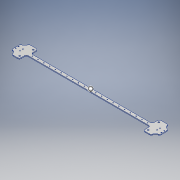
# Autodesk Inventor part: XY_Plate
Saved by Autodesk Inventor 2019 (Build 230136000, 136)
## iProperties
Created: 2018-10-13
Part Number: XY_Plate
Material: Aluminum 6061
Document SubType Name: Sheet Metal
Designer: Ax
Density: 2.7 g/cm^3
Sheet Metal Rule: Default_mm
Appearance: Aluminum - Flat
Mass: 72.1012 g
Surface Area: 222.709 cm^2
Volume: 26.7041 cm^3
Flat Pattern Width: 6 cm
Flat Pattern Length: 51.2 cm
Flat Pattern Area: 307.2 cm^2
Sheet Metal Width: 60.000 mm
Sheet Metal Length: 512.000 mm
Sheet Metal Area: 30720.000 mm^2
Author: Ax
Autodesk Inventor part; units mm, degrees
ref_plane "YZ Plane" through (0, 0, 0) normal (1, 0, 0) x (0, 1, 0)
ref_plane "XZ Plane" through (0, 0, 0) normal (0, 1, 0) x (-1, 0, 0)
ref_plane "XY Plane" through (0, 0, 0) normal (0, 0, 1) x (1, 0, 0)
sketch "Sketch1" plane through (0, 0, 0) normal (0, 0, 1) x (1, 0, 0)
  line L0 (0, 5.5) -> (-215, 5.5)
  line L1 (-215, -5.5) -> (0, -5.5)
  line L2 (0, -5.5) -> (0, 5.5)
  line L3 (0, 0) -> (-256, 0) construction
  line L4 (-256, 30) -> (-215, 30)
  line L5 (-215, -30) -> (-256, -30)
  line L6 (-256, -30) -> (-256, 30)
  line L7 (-215, 30) -> (-215, 5.5)
  line L8 (-215, -5.5) -> (-215, -30)
  dimension "d0" = 11
  dimension "d1" = 215
  dimension "d2" = 60
  dimension "d3" = 41
  measures "d0" distance of L1.end L0.start
  measures "d1" distance of L1.start L1.end
  measures "d2" distance of L5.end L4.start
  measures "d3" distance of L5.start L5.end
extrude "Plate1" add sketch "Sketch1" along normal blind 3
sketch "Sketch2" plane through (0, 0, 3) normal (0, 0, 1) x (1, 0, 0)
  line L0 (-256, 30) -> (-256, -30) projected
  arc A0 (-256, 15) -> (-241, 30) centre (-256, 30) ccw
  line L1 (-256, -30) -> (-215, -30) projected
  arc A1 (-241, -30) -> (-256, -15) centre (-256, -30) ccw
  line L2 (-256, 30) -> (-215, 30) projected
  line L3 (-215, -30) -> (-256, -30) projected
  line L4 (-256, -30) -> (-256, 30) projected
  line L5 (-256, 0) -> (-215, 0) construction
  point P0 (0, 0)
  dimension "d5" = 30
  constraints: 4 point on circle, 4 point on line, 2 centre point, 2 end point, 1 coincident, 1 horizontal, 1 midpoint, 1 symmetric about line
  measures "d5" distance of A1.end A0.start
extrude "Extrusion1" cut sketch "Sketch2" against normal through all
sketch "Sketch3" plane through (0, 0, 3) normal (0, 0, 1) x (1, 0, 0)
  line L0 (-252.5, -5) -> (-237.5, -5) construction
  line L1 (-237.5, -5) -> (-237.5, 5) construction
  line L2 (-237.5, 5) -> (-252.5, 5) construction
  line L3 (-252.5, 5) -> (-252.5, -5) construction
  line L4 (-252.5, -5) -> (-237.5, 5) construction
  line L5 (-237.5, -5) -> (-252.5, 5) construction
  line L6 (-256, -15) -> (-256, 15) construction
  line L7 (-256, 0) -> (-245, 0) construction
  circle A0 centre (-237.5, 5) radius 1.6
  circle A1 centre (-237.5, -5) radius 1.6
  circle A2 centre (-252.5, -5) radius 1.6
  circle A3 centre (-252.5, 5) radius 1.6
  point P0 (0, 0)
  point P1 (-255, -13.1181)
  point P2 (-255, 13.1181)
  dimension "d10" = 3.5
  dimension "d11" = 15
  dimension "d12" = 10
  dimension "d13" = 3.2
  constraints: 14 end point, 4 centre point, 4 coincident, 3 equal radius, 2 horizontal, 2 midpoint, 2 parallel, 1 perpendicular, 2 other
  measures "d11" distance of L0.start L0.end
  measures "d12" distance of L0.end L1.end
  measures "d13" diameter of A0
extrude "Extrusion2" cut sketch "Sketch3" against normal through all
mirror "Mirror2" about plane through (0, 0, 0) normal (1, 0, 0) of "Plate1", "Extrusion1", "Extrusion2"
thicken "Thicken1" operation add thickness 5 both sides no extend neighbours yes toward (1, 0, 0) faces at (-215, 13.6667, 2)
thicken "Thicken3" operation add thickness 5 both sides no extend neighbours yes toward (-1, 0, 0) faces at (215, 13.6667, 2)
sketch "Sketch4" plane through (0, 0, 0) normal (0, 0, -1) x (-1, 0, 0)
  circle A0 centre (0, 0) radius 1.25
  dimension "d18" = 2.5
  constraints: 1 centre point, 1 coincident
  measures "d18" diameter of A0
hole "Hole1" at (0, 0, 0) direction (0, 0, 1) diameter 2.459 end through all thread size "M3x0.5" class "6H" standard "ISO Metric profile"
pattern_linear "Rectangular Pattern1" count 21 spacing 20 along (1, 0, 0) of "Hole1" first direction both ways yes
sketch "Sketch5" plane through (0, 0, 0) normal (0, 0, -1) x (-1, 0, 0)
  circle A0 centre (-222.5, -21) radius 2.6
  line L0 (-241, 30) -> (-215, 30) construction
  line L1 (-241, -30) -> (-215, -30) construction
  line L2 (-224, 0) -> (-224, 0) construction
  line L3 (-215, -30) -> (-215, -5.5) projected
  circle A1 centre (-217.5, 21) radius 2.6
  line L4 (-210, 5.5) -> (-210, 30) projected
  point P0 (0, 0)
  point P1 (-224, 0)
  dimension "d26" = 5.2
  dimension "d42" = 9
  dimension "d45" = 7.5
  dimension "d47" = 9
  dimension "d56" = 7.5
  constraints: 2 centre point, 2 end point, 1 equal radius, 1 horizontal, 1 midpoint
  measures "d26" diameter of A0
  measures "d42" distance from line of L1 A0.centre
  measures "d45" distance from line of L3 A0.centre
  measures "d47" distance from line of L0 A1.centre
  measures "d56" distance from line of A1.centre L4
extrude "Cut2" cut sketch "Sketch5" against normal blind 3
sketch "Sketch6" plane through (0, 0, 3) normal (0, 0, 1) x (1, 0, 0)
  circle A0 centre (-222.5, -21) radius 2.6
  line L0 (-215, -5.5) -> (-215, -30) projected
  circle A1 centre (-217.5, 21) radius 2.6
  line L1 (-210, 30) -> (-210, 5.5) projected
  line L2 (-215, -30) -> (-241, -30) projected
  line L3 (-241, 30) -> (-210, 30) projected
  point P0 (0, 0)
  dimension "d37" = 5.2
  dimension "d49" = 7.5
  dimension "d50" = 9
  dimension "d51" = 7.5
  dimension "d52" = 9
  constraints: 2 centre point, 1 equal radius
  measures "d37" diameter of A1
  measures "d49" distance from line of L0 A0.centre
  measures "d50" distance from line of L2 A0.centre
  measures "d51" distance from line of L1 A1.centre
  measures "d52" distance from line of L3 A1.centre
extrude "Cut3" cut sketch "Sketch6" against normal blind 3
fillet "Corner Round1" radius 6 16 edges at (215, -30, 1.5) (241, -30, 1.5) (256, -15, 1.5) (241, 30, 1.5) (210, 30, 1.5) (210, 5.5, 1.5) (215, -5.5, 1.5) (256, 15, 1.5) (-215, -30, 1.5) (-215, -5.5, 1.5) (-210, 5.5, 1.5) (-210, 30, 1.5) (-241, 30, 1.5) (-256, 15, 1.5) (-256, -15, 1.5) (-241, -30, 1.5)
equation "\"d27\" = Thickness"
equation "\"d38\" = Thickness"
equation "\"d32\" = Thickness"
equation "\"CornerReliefSize\" = 4 * Thickness"
equation "\"TransitionRadius\" = BendRadius"
equation "\"JacobiRadiusSize\" = BendRadius"
equation "\"d4\" = BendRadius"
equation "\"Thickness\" = 3"
equation "\"BendRadius\" = 0.8"
body "Solid1"
